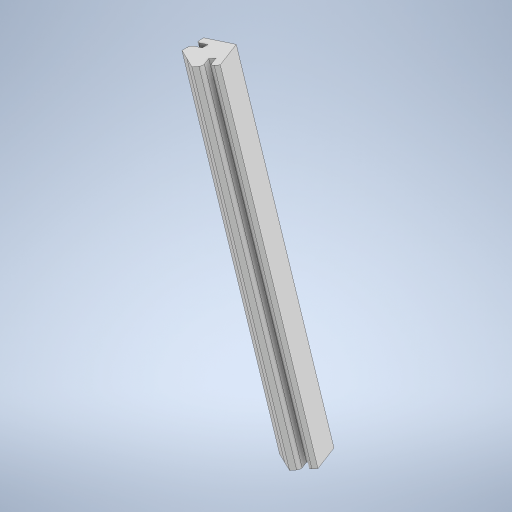
# Autodesk Inventor part: Pieza1
Saved by Autodesk Inventor 2024 (Build 280153000, 153)
## iProperties
Created: 2025-08-12
Part Number: Pieza1
Material: Genérico
Document SubType Name: Modeling
Designer: sergi
Density: 1 g/cm^3
Appearance: Valor por defecto
Author: sergi
Autodesk Inventor part; units mm, degrees
sketch "Boceto1" plane through (0, 0, 0) normal (0, 0, 1) x (1, 0, 0)
  line L0 (-5.9, 8.1207) -> (5.9, 8.1207)
  line L1 (5.9, 8.1207) -> (9.5464, -3.1018)
  line L2 (9.5464, -3.1018) -> (0, -10.0377)
  line L3 (0, -10.0377) -> (-9.5464, -3.1018)
  line L4 (-9.5464, -3.1018) -> (-5.9, 8.1207)
  line L5 (0, 0) -> (-16.2413, 0)
  line L6 (-16.2413, 0) -> (-16.2413, 16.2413)
  line L7 (-16.2413, 16.2413) -> (0, 16.2413)
  line L8 (0, 16.2413) -> (0, 0)
  line L9 (0, 8.1207) -> (-16.2413, 16.2413)
  dimension "d0" = 11.8
  dimension "d1" = 26.279
  dimension "d2" = 26.565
  constraints: 20 end point, 2 horizontal, 2 midpoint, 2 parallel, 2 perpendicular, 1 coincident, 11 other
  measures "d0" distance of L0.start L0.end
  measures "d1" distance from line of L2.end L7
  measures "d2" angle of L0 L9
extrude "Extrusión1" add sketch "Boceto1" along normal blind 26.279 draft 26.57 contours L0 L8 L5 L4 | L0 L1 L2 L3 L4 L5 L8
sketch "Boceto2" plane through (0, 0, 26.279) normal (0, 0, 1) x (1, 0, 0)
  line L0 (0, 10.0377) -> (9.5464, 3.1018)
  line L1 (9.5464, 3.1018) -> (5.9, -8.1207)
  line L2 (5.9, -8.1207) -> (-5.9, -8.1207)
  line L3 (-5.9, -8.1207) -> (-9.5464, 3.1018)
  line L4 (-9.5464, 3.1018) -> (0, 10.0377)
  point P0 (0, 0)
  point P1 (0, 0)
  dimension "d5" = 11.8
  constraints: 10 end point, 1 coincident, 1 horizontal, 11 other
  measures "d5" distance of L3.end L0.start
extrude "Extrusión2" cut sketch "Boceto2" against normal through all draft 26.57 keep common part
sketch "Boceto3" plane through (-9.5464, -3.1018, 0) normal (-0.8506141, 0.2763813, -0.4472908) x (-0.4253989, 0.1382205, 0.8943886)
  line L0 (18.1587, 5.9) -> (11.2234, -3.6473) projected
  line L1 (11.2234, 15.4473) -> (18.1587, 5.9) projected
  line L2 (0, 11.8) -> (11.2234, 15.4473) projected
  line L3 (0, 11.8) -> (0, 0) projected
  line L4 (0, 0) -> (11.2234, -3.6473) projected
  line L5 (1.1, 0.7992) -> (1.1, 11.0008)
  line L6 (1.1, 11.0008) -> (10.8032, 14.1541)
  line L7 (10.8032, 14.1541) -> (16.7991, 5.9)
  line L8 (16.7991, 5.9) -> (10.8032, -2.3541)
  line L9 (10.8032, -2.3541) -> (1.1, 0.7992)
  point P0 (-3.6323, 5.9)
  dimension "d8" = 1.1
  constraints: 10 end point, 4 other
  measures "d8" distance between parallel lines of L3 L5
extrude "Extrusión3" cut sketch "Boceto3" against normal blind 20 contours L5 L6 L7 L8 L9
sketch "Boceto4" plane through (-9.5464, -3.1018, 0) normal (-0.5257084, -0.7235755, -0.4472908) x (0.809017, -0.5877853, 0)
  line L0 (-8.9695, 3.2885) -> (8.0428, 8.8171) projected
  line L1 (5.9, 18.1587) -> (15.4473, 11.2234) projected
  line L2 (-3.6473, 11.2234) -> (5.9, 18.1587) projected
  line L3 (0, 0) -> (-3.6473, 11.2234) projected
  line L4 (0, 0) -> (11.8, 0) projected
  line L5 (11.8, 0) -> (15.4473, 11.2234) projected
  line L6 (14.1541, 10.8032) -> (5.9, 16.7991)
  line L7 (5.9, 16.7991) -> (-2.3541, 10.8032)
  line L8 (-2.3541, 10.8032) -> (0.7992, 1.1)
  line L9 (0.7992, 1.1) -> (11.0008, 1.1)
  line L10 (11.0008, 1.1) -> (14.1541, 10.8032)
  point P0 (5.9, -3.6323)
  point P1 (12.4344, 10.2443)
  dimension "d11" = 1.1
  constraints: 10 end point, 4 other
  measures "d11" distance between parallel lines of L5 L10
extrude "Extrusión4" cut sketch "Boceto4" against normal blind 20 contours L10 L9 L8 L7 L6
sketch "Boceto5" plane through (0, 0, 0) normal (0, 0, -1) x (-1, 0, 0)
  line L0 (0, -10.0377) -> (-9.5464, -3.1018) projected
  line L1 (9.5464, -3.1018) -> (0, -10.0377) projected
  line L2 (5.9, 8.1207) -> (9.5464, -3.1018) projected
  line L3 (-5.9, 8.1207) -> (5.9, 8.1207) projected
  line L4 (-9.5464, -3.1018) -> (-5.9, 8.1207) projected
  line L5 (-8.2533, -2.6817) -> (0, -8.678)
  line L6 (0, -8.678) -> (8.2533, -2.6817)
  line L7 (8.2533, -2.6817) -> (5.1008, 7.0207)
  line L8 (5.1008, 7.0207) -> (-5.1008, 7.0207)
  line L9 (-5.1008, 7.0207) -> (-8.2533, -2.6817)
  point P0 (0, 0)
  dimension "d14" = 1.1
  constraints: 10 end point, 4 other
  measures "d14" distance between parallel lines of L0 L5
extrude "Extrusión5" cut sketch "Boceto5" against normal blind 20 contours L9 L8 L7 L6 L5
sketch "Boceto6" plane through (-15.4479, 5.0193, 16.2409) normal (-0.8506141, -0.2763813, 0.4472908) x (0.5000781, -0.1624852, 0.8506)
  line L0 (15.4481, -11.2223) -> (11.8011, 0) projected
  line L1 (11.8011, 0) -> (0, 0) projected
  line L2 (0, 0) -> (-3.645, -11.2234) projected
  line L3 (-3.645, -11.2234) -> (5.9015, -18.1598) projected
  line L4 (15.4481, -11.2223) -> (5.9015, -18.1598) projected
  line L5 (-2.352, -10.8032) -> (0.7993, -1.1)
  line L6 (0.7993, -1.1) -> (11.002, -1.1)
  line L7 (11.002, -1.1) -> (14.155, -10.8022)
  line L8 (14.155, -10.8022) -> (5.9014, -16.8)
  line L9 (5.9014, -16.8) -> (-2.352, -10.8032)
  point P0 (-5.2738, -11.7527)
  dimension "d0" = 11.8
  dimension "d1" = 26.279
  dimension "d2" = 26.565
  dimension "d17" = 1.1
  constraints: 10 end point, 4 other
  measures "d17" distance between parallel lines of L2 L5
extrude "Extrusión6" cut sketch "Boceto6" against normal blind 20 contours L5 L6 L7 L8 L9
sketch "Boceto7" plane through (-9.5464, 3.1018, 26.279) normal (-0.5257084, 0.7235755, 0.4472908) x (0.809017, 0.5877853, 0)
  line L0 (8.0428, 11.1714) -> (9.626, 8.4786) projected
  line L1 (13.1449, 14.4423) -> (8.0428, 7.4219) projected
  line L2 (15.4473, 11.2234) -> (5.9, 18.1587) projected
  line L3 (5.9, 18.1587) -> (-3.6473, 11.2234) projected
  line L4 (0, 0) -> (-3.6473, 11.2234) projected
  line L5 (0, 0) -> (11.8, 0) projected
  line L6 (11.8, 0) -> (15.4473, 11.2234) projected
  line L7 (-2.3541, 10.8032) -> (5.9, 16.7991)
  line L8 (5.9, 16.7991) -> (14.1541, 10.8032)
  line L9 (14.1541, 10.8032) -> (11.0008, 1.1)
  line L10 (11.0008, 1.1) -> (0.7992, 1.1)
  line L11 (0.7992, 1.1) -> (-2.3541, 10.8032)
  point P0 (5.9, 19.8713)
  dimension "d20" = 1.1
  constraints: 10 end point, 4 other
  measures "d20" distance between parallel lines of L3 L7
extrude "Extrusión7" cut sketch "Boceto7" against normal blind 20 contours L7 L8 L9 L10 L11
sketch "Boceto8" plane through (-5.9, 8.1207, 0) normal (0, 0.8943886, -0.4472908) x (1, 0, 0)
  line L0 (15.4473, -11.2234) -> (5.9, -18.1587) projected
  line L1 (11.8, 0) -> (15.4473, -11.2234) projected
  line L2 (11.8, 0) -> (0, 0) projected
  line L3 (0, 0) -> (-3.6473, -11.2234) projected
  line L4 (5.9, -18.1587) -> (-3.6473, -11.2234) projected
  line L5 (0.7992, -1.1) -> (11.0008, -1.1)
  line L6 (11.0008, -1.1) -> (14.1541, -10.8032)
  line L7 (14.1541, -10.8032) -> (5.9, -16.7991)
  line L8 (5.9, -16.7991) -> (-2.3541, -10.8032)
  line L9 (-2.3541, -10.8032) -> (0.7992, -1.1)
  point P0 (5.9, 3.6323)
  dimension "d23" = 1.1
  constraints: 10 end point, 4 other
  measures "d23" distance between parallel lines of L2 L5
extrude "Extrusión8" cut sketch "Boceto8" against normal blind 20 contours L5 L6 L7 L8 L9
sketch "Boceto9" plane through (0, 0, 26.279) normal (0, 0, 1) x (1, 0, 0)
  line L0 (5.9, -8.1207) -> (-5.9, -8.1207) projected
  line L1 (9.5464, 3.1018) -> (5.9, -8.1207) projected
  line L2 (0, 10.0377) -> (9.5464, 3.1018) projected
  line L3 (-9.5464, 3.1018) -> (0, 10.0377) projected
  line L4 (-5.9, -8.1207) -> (-9.5464, 3.1018) projected
  line L5 (-8.2533, 2.6817) -> (0, 8.678)
  line L6 (0, 8.678) -> (8.2533, 2.6817)
  line L7 (8.2533, 2.6817) -> (5.1008, -7.0207)
  line L8 (5.1008, -7.0207) -> (-5.1008, -7.0207)
  line L9 (-5.1008, -7.0207) -> (-8.2533, 2.6817)
  point P0 (0, 0)
  dimension "d26" = 1.1
  constraints: 10 end point, 4 other
  measures "d26" distance between parallel lines of L4 L9
extrude "Extrusión9" cut sketch "Boceto9" against normal blind 20 contours L5 L6 L7 L8 L9
sketch "Boceto10" plane through (0, 10.0377, 26.279) normal (0.5257084, 0.7235755, 0.4472908) x (0.809017, -0.5877853, 0)
  line L0 (15.4473, 11.2234) -> (5.9, 18.1587) projected
  line L1 (5.9, 18.1587) -> (-3.6473, 11.2234) projected
  line L2 (0, 0) -> (-3.6473, 11.2234) projected
  line L3 (0, 0) -> (11.8, 0) projected
  line L4 (11.8, 0) -> (15.4473, 11.2234) projected
  line L5 (-2.3541, 10.8032) -> (5.9, 16.7991)
  line L6 (5.9, 16.7991) -> (14.1541, 10.8032)
  line L7 (14.1541, 10.8032) -> (11.0008, 1.1)
  line L8 (11.0008, 1.1) -> (0.7992, 1.1)
  line L9 (0.7992, 1.1) -> (-2.3541, 10.8032)
  point P0 (5.9, 19.8713)
  dimension "d29" = 1.1
  constraints: 10 end point, 4 other
  measures "d29" distance between parallel lines of L1 L5
extrude "Extrusión10" cut sketch "Boceto10" against normal blind 20 contours L5 L6 L7 L8 L9
sketch "Boceto11" plane through (9.5464, -3.1018, 0) normal (0.8506141, 0.2763813, -0.4472908) x (-0.4253989, -0.1382205, -0.8943886)
  line L0 (-11.2234, -3.6473) -> (-18.1587, 5.9) projected
  line L1 (0, 0) -> (-11.2234, -3.6473) projected
  line L2 (0, 0) -> (0, 11.8) projected
  line L3 (0, 11.8) -> (-11.2234, 15.4473) projected
  line L4 (-18.1587, 5.9) -> (-11.2234, 15.4473) projected
  line L5 (-10.8032, 14.1541) -> (-1.1, 11.0008)
  line L6 (-1.1, 11.0008) -> (-1.1, 0.7992)
  line L7 (-1.1, 0.7992) -> (-10.8032, -2.3541)
  line L8 (-10.8032, -2.3541) -> (-16.7991, 5.9)
  line L9 (-16.7991, 5.9) -> (-10.8032, 14.1541)
  point P0 (3.6323, 5.9)
  dimension "d32" = 1.1
  constraints: 10 end point, 4 other
  measures "d32" distance between parallel lines of L3 L5
extrude "Extrusión11" cut sketch "Boceto11" against normal blind 20 contours L5 L6 L7 L8 L9
sketch "Boceto12" plane through (0, -10.0377, 0) normal (0.5257084, -0.7235755, -0.4472908) x (0.809017, 0.5877853, 0)
  line L0 (5.9, 18.1587) -> (15.4473, 11.2234) projected
  line L1 (-3.6473, 11.2234) -> (5.9, 18.1587) projected
  line L2 (0, 0) -> (-3.6473, 11.2234) projected
  line L3 (0, 0) -> (11.8, 0) projected
  line L4 (11.8, 0) -> (15.4473, 11.2234) projected
  line L5 (14.1541, 10.8032) -> (5.9, 16.7991)
  line L6 (5.9, 16.7991) -> (-2.3541, 10.8032)
  line L7 (-2.3541, 10.8032) -> (0.7992, 1.1)
  line L8 (0.7992, 1.1) -> (11.0008, 1.1)
  line L9 (11.0008, 1.1) -> (14.1541, 10.8032)
  point P0 (5.9, -3.6323)
  dimension "d35" = 1.1
  constraints: 10 end point, 4 other
  measures "d35" distance between parallel lines of L4 L9
extrude "Extrusión12" cut sketch "Boceto12" against normal blind 20 contours L9 L8 L7 L6 L5
sketch "Boceto13" plane through (-5.9, -8.1207, 26.279) normal (0, -0.8943886, 0.4472908) x (1, 0, 0)
  line L0 (5.9, -18.1587) -> (15.4473, -11.2234) projected
  line L1 (11.8, 0) -> (15.4473, -11.2234) projected
  line L2 (11.8, 0) -> (0, 0) projected
  line L3 (0, 0) -> (-3.6473, -11.2234) projected
  line L4 (-3.6473, -11.2234) -> (5.9, -18.1587) projected
  line L5 (14.1541, -10.8032) -> (5.9, -16.7991)
  line L6 (5.9, -16.7991) -> (-2.3541, -10.8032)
  line L7 (-2.3541, -10.8032) -> (0.7992, -1.1)
  line L8 (0.7992, -1.1) -> (11.0008, -1.1)
  line L9 (11.0008, -1.1) -> (14.1541, -10.8032)
  point P0 (5.9, -19.8713)
  dimension "d38" = 1.1
  constraints: 10 end point, 4 other
  measures "d38" distance between parallel lines of L1 L9
extrude "Extrusión13" cut sketch "Boceto13" against normal blind 20 contours L5 L6 L7 L8 L9
sketch "Boceto14" plane through (5.9, -8.1207, 26.279) normal (0.8506141, -0.2763813, 0.4472908) x (0.4253989, -0.1382205, -0.8943886)
  line L0 (11.2234, -3.6473) -> (18.1587, 5.9) projected
  line L1 (18.1587, 5.9) -> (11.2234, 15.4473) projected
  line L2 (0, 11.8) -> (11.2234, 15.4473) projected
  line L3 (0, 11.8) -> (0, 0) projected
  line L4 (0, 0) -> (11.2234, -3.6473) projected
  line L5 (10.8032, 14.1541) -> (16.7991, 5.9)
  line L6 (16.7991, 5.9) -> (10.8032, -2.3541)
  line L7 (10.8032, -2.3541) -> (1.1, 0.7992)
  line L8 (1.1, 0.7992) -> (1.1, 11.0008)
  line L9 (1.1, 11.0008) -> (10.8032, 14.1541)
  point P0 (19.8713, 5.9)
  dimension "d41" = 1.1
  constraints: 10 end point, 4 other
  measures "d41" distance between parallel lines of L1 L5
extrude "Extrusión14" cut sketch "Boceto14" against normal blind 20 contours L5 L6 L7 L8 L9
ref_plane "Plano de trabajo1" through (0, 0, 0.25) normal (0, 0, -1) x (-1, 0, 0)
sketch "Boceto15" plane through (0, 0, 0.25) normal (0, 0, -1) x (-1, 0, 0)
  line L0 (5.1008, 7.0207) -> (8.2533, -2.6817) projected
  line L1 (8.2533, -2.6817) -> (0, -8.678) projected
  line L2 (0, -8.678) -> (-8.2533, -2.6817) projected
  line L3 (-8.2533, -2.6817) -> (-5.1008, 7.0207) projected
  line L4 (-5.1008, 7.0207) -> (5.1008, 7.0207) projected
  line L5 (0, -10.0377) -> (-9.5464, -3.1018) projected
  line L6 (9.5464, -3.1018) -> (0, -10.0377) projected
  line L7 (5.9, 8.1207) -> (9.5464, -3.1018) projected
  line L8 (-5.9, 8.1207) -> (5.9, 8.1207) projected
  line L9 (-9.5464, -3.1018) -> (-5.9, 8.1207) projected
  line L10 (8.7235, -2.8344) -> (0, -9.1724)
  line L11 (0, -9.1724) -> (-8.7235, -2.8344)
  line L12 (-8.7235, -2.8344) -> (-5.3914, 7.4207)
  line L13 (-5.3914, 7.4207) -> (5.3914, 7.4207)
  line L14 (5.3914, 7.4207) -> (8.7235, -2.8344)
  point P0 (0, 0)
  dimension "d45" = 0.7
  constraints: 10 end point, 4 other
  measures "d45" distance between parallel lines of L7 L14
extrude "Extrusión15" cut sketch "Boceto15" against normal blind 0.18 contours L0 L1 L2 L3 L4 | L10 L11 L12 L13 L14
ref_plane "Plano de trabajo2" through (5.9, 8.1207, 0) normal (-0.809017, 0.5877853, 0) x (-0.5877853, -0.809017, 0)
ref_plane "Plano de trabajo3" through (5.9, 8.1207, 0) normal (0.8090319, 0.2629018, 0.52569) x (-0.5877647, 0.3618726, 0.7235889)
ref_plane "Plano de trabajo4" through (5.9, 8.1207, 0) normal (-0.0000133, -0.8506708, -0.5256987) x (0.5257906, -0.4471727, 0.7235889)
ref_plane "Plano de trabajo5" through (9.5464, -3.1018, 0) normal (0.309017, 0.9510565, 0) x (-0.9510565, 0.309017, 0)
ref_plane "Plano de trabajo6" through (9.5464, -3.1018, 0) normal (0.5000391, -0.688194, 0.52569) x (0.162532, 0.6708222, 0.7235889)
ref_plane "Plano de trabajo7" through (9.5464, -3.1018, 0) normal (-0.8090402, -0.2628591, -0.5256987) x (-0.2628083, -0.6382405, 0.7235889)
split "Dividir1" plane through (9.5464, -3.1018, 0) removes the side toward (0.5000391, -0.688194, 0.52569)
split "Dividir2" plane through (9.5464, -3.1018, 0) removes the side toward (-0.309017, -0.9510565, 0)
split "Dividir3" plane through (5.9, 8.1207, 0) removes the side toward (0.0000133, 0.8506708, 0.5256987)
split "Dividir4" plane through (5.9, 8.1207, 0) removes the side toward (-0.809017, 0.5877853, 0)
ref_plane "Plano de trabajo9" through (7.306, -0.787, 0.5104) normal (0.4999651, 0.1624485, -0.8506735) x (-0.309017, 0.9510565, 0)
ref_plane "Plano de trabajo8" through (7.606, -0.6896, 0) normal (0.4999651, 0.1624485, -0.8506735) x (-0.309017, 0.9510565, 0)
split "Dividir5" plane through (7.306, -0.787, 0.5104) removes the side toward (-0.4999651, -0.1624485, 0.8506735)
ref_plane "Plano de trabajo10" through (9.5464, -3.1018, 0) normal (-0.8090468, -0.2628753, -0.5256803) x (-0.309017, 0.9510565, 0)
split "Dividir6" plane through (9.5464, -3.1018, 0) removes the side toward (0.8090468, 0.2628753, 0.5256803)
fillet "Empalme1" radius 0.1 2 edges at (6.677, 2.1695, 0.43) (6.677, 2.1695, 0.25)
mirror "Simetría1" about plane through (9.5464, -3.1018, 0) normal (-0.8090468, -0.2628753, -0.5256803)
ref_plane "Plano de trabajo11" through (9.7674, -2.1897, 0.9838) normal (-0.309017, 0.9510565, 0) x (-0.8506, -0.2763767, 0.4473204)
ref_plane "Plano de trabajo12" through (6.6149, 7.5126, 0.9838) normal (-0.309017, 0.9510565, 0) x (-0.8506, -0.2763767, 0.4473204)
split "Dividir7" plane through (9.7674, -2.1897, 0.9838) removes the side toward (0.309017, -0.9510565, 0)
split "Dividir8" plane through (6.6149, 7.5126, 0.9838) removes the side toward (-0.309017, 0.9510565, 0)
equation "\"d3\" = d1"
